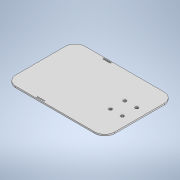
# Autodesk Inventor part: podstawa
Saved by Autodesk Inventor 2020 (Build 240168000, 168)
## iProperties
Created: 2022-04-08
Part Number: podstawa
Material: Ogólny
Document SubType Name: Modeling
Designer: aleks
Density: 1 g/cm^3
Appearance: Domyślna
Author: aleks
Autodesk Inventor part; units mm, degrees
ref_plane "YZ Plane" through (0, 0, 0) normal (1, 0, 0) x (0, 1, 0)
ref_plane "XZ Plane" through (0, 0, 0) normal (0, 1, 0) x (-1, 0, 0)
ref_plane "XY Plane" through (0, 0, 0) normal (0, 0, 1) x (1, 0, 0)
sketch "Szkic1" plane through (0, 0, 0) normal (0, 1, 0) x (-1, 0, 0)
  line L0 (0, 0) -> (-200, 0)
  line L1 (-200, 0) -> (-200, 140)
  line L2 (-200, 140) -> (0, 140)
  line L3 (0, 140) -> (0, 0)
  dimension "d0" = 200
  dimension "d1" = 140
  constraints: 8 end point, 2 parallel, 1 horizontal, 1 perpendicular
  measures "d0" distance of L1.end L2.end
  measures "d1" distance of L0.end L1.end
extrude "Wyciągnięcie proste1" add sketch "Szkic1" along normal blind 3
sketch "Szkic2" plane through (0, 3, 0) normal (0, 1, 0) x (1, 0, 0)
  line L0 (0, 0) -> (50, 0)
  line L1 (200, 0) -> (0, 0) projected
  line L2 (50, 0) -> (60, 0)
  line L3 (60, 0) -> (60, -2)
  line L4 (60, -2) -> (75, -2)
  line L5 (75, -2) -> (75, -4)
  line L6 (75, -4) -> (60, -4)
  line L7 (60, -4) -> (60, -2)
  line L8 (0, 0) -> (0, -140) projected
  line L9 (0, -70) -> (200, -70)
  line L10 (200, -140) -> (200, 0) projected
  line L11 (60, -140) -> (60, -138)
  line L12 (60, -138) -> (75, -138)
  line L13 (75, -138) -> (75, -136)
  line L14 (75, -136) -> (60, -136)
  line L15 (60, -136) -> (60, -138)
  dimension "d4" = 50
  dimension "d5" = 10
  dimension "d6" = 2
  dimension "d7" = 15
  dimension "d8" = 2
  constraints: 26 end point, 5 symmetric about line, 2 midpoint, 2 parallel, 2 perpendicular, 2 point on line, 1 horizontal
  measures "d4" distance of L0.start L0.end
  measures "d5" distance of L0.end L2.end
  measures "d6" distance of L2.end L3.end
  measures "d7" distance of L5.end L6.end
  measures "d8" distance of L4.end L5.end
extrude "Wyciągnięcie proste2" cut sketch "Szkic2" against normal blind 3 contours L4 L5 L6 L7 | L15 L14 L13 L12
sketch "Szkic3" plane through (0, 3, 0) normal (0, 1, 0) x (1, 0, 0)
  line L0 (200, -140) -> (200, 0) projected
  line L1 (0, -140) -> (200, -140) projected
  line L2 (200, 0) -> (180, 0)
  line L3 (180, 0) -> (180, -140)
  line L4 (180, -140) -> (200, -140)
  line L5 (200, -140) -> (200, 0)
  line L6 (180, -70) -> (180, -53)
  line L7 (180, -53) -> (180, -55.5)
  circle A0 centre (180, -55.5) radius 3
  line L8 (180, -55.5) -> (156, -55.5)
  circle A1 centre (156, -55.5) radius 3
  line L9 (200, -70) -> (129.0719, -70)
  circle A2 centre (180, -84.5) radius 3
  circle A3 centre (156, -84.5) radius 3
  point P0 (0, 0)
  dimension "d11" = 20
  dimension "d12" = 17
  dimension "d13" = 2.5
  dimension "d14" = 6
  dimension "d15" = 24
  dimension "d16" = 6
  constraints: 16 end point, 4 centre point, 3 horizontal, 3 point on line, 2 coincident, 2 midpoint, 2 parallel, 2 symmetric about line, 1 perpendicular, 2 other
  measures "d11" distance of L4.end L3.end
  measures "d12" distance of L6.start L6.end
  measures "d13" distance of L6.end L7.end
  measures "d14" diameter of A0
  measures "d15" distance of L8.start L8.end
  measures "d16" diameter of A1
extrude "Wyciągnięcie proste3" cut sketch "Szkic3" against normal blind 3 contours A1 | A2 L3 | L3 A2 | A0 L8 L3 | L3 A0 | L3 L8 A0 | A3
fillet "Zaokrąglenie1" radius 20 4 edges at (0, 1.5, 140) (0, 1.5, 0) (200, 1.5, 0) (200, 1.5, 140)
